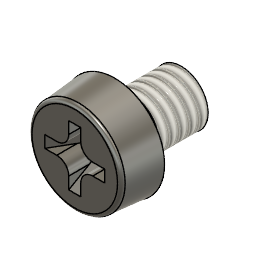
newest macropad desing (Autodesk Fusion 360 archive; units mm, degrees)
design "Cheese Head Screw BS EN ISO 7048 - M2.5 x 3 - H Steel 4.6 Plain"
description: Cheese Head Screw BS EN ISO 7048 - M2.5 x 3 - H
part number: BS EN ISO 7048 - H - M2.5 x 3 Steel 4.6 Plain
Autodesk Fusion 360 part; units mm, degrees
sketch "Sketch1" plane through (0, 0, 0) normal (0, 1, 0) x (1, 0, 0)
  line L0 (0, -1.8) -> (0, 3)
  line L1 (-2.25, 0) -> (-2.0925, -1.8)
  line L2 (-2.25, 0) -> (-1.0925, 0)
  line L3 (0, 3) -> (-1.25, 3)
  line L4 (-1.25, 3) -> (-1.25, 0.9)
  line L5 (-1.25, 0.9) -> (-1.0925, 0.3122)
  line L6 (-1.0925, 0.3122) -> (-1.0925, 0)
  line L7 (0, -1.8) -> (-2.0925, -1.8)
  dimension "d13" = 5
  dimension "d14" = 4.5
  dimension "d18" = 2.5
  dimension "d56" = 3
  dimension "d65" = 15
  dimension "d67" = 1.8
  dimension "d71" = 2.185
  dimension "d77" = 0.9
  constraint vertical L0
  constraint coincident origin L0
  constraint coincident origin L2
  constraint perpendicular L0 L3
  constraint coincident L2.end L6.end
  constraint perpendicular L0 L7
  measures "d13" angle of L0 L1
  measures "d56" distance of L2 L3
  measures "d65" angle of L5 L6
  measures "d67" distance of L1.start L7
  measures "d77" distance of L2 L4.end
revolve "Revolve1" add sketch "Sketch1" angle 360 about axis through (0, 0, 1.8) along (0, 0, -1) makes body 1
fillet "Fillet3" radius 0.18 1 edges at (-1.9509, 0.7567, 1.8) on bodies 1
fillet "Fillet2" radius 0.1 1 edges at (-1.0186, 0.3951, 0) on bodies 1
sketch "Sketch2" plane through (0, 0, 1.8) normal (0, 0, 1) x (1, 0, 0)
  line L0 (-0.27, 0.27) -> (-1.35, 0.27)
  line L1 (-1.35, 0.27) -> (-1.35, -0.27)
  line L2 (-1.35, -0.27) -> (-0.27, -0.27)
  line L3 (-0.27, -0.27) -> (-0.27, -1.35)
  line L4 (-0.27, -1.35) -> (0.27, -1.35)
  line L5 (0.27, -1.35) -> (0.27, -0.27)
  line L6 (0.27, -0.27) -> (1.35, -0.27)
  line L7 (1.35, -0.27) -> (1.35, 0.27)
  line L8 (1.35, 0.27) -> (0.27, 0.27)
  line L9 (0.27, 0.27) -> (0.27, 1.35)
  line L10 (0.27, 1.35) -> (-0.27, 1.35)
  line L11 (-0.27, 1.35) -> (-0.27, 0.27)
  dimension "d81" = 360
  dimension "d83" = 0.54
  dimension "d84" = 2.7
  constraint horizontal L0
  constraint perpendicular L0 L1
  constraint vertical L0.start L2.end
  constraint coincident L2.end L3.start
  measures "d83" distance of L0 L2
  measures "d84" distance of L1 L6.end
extrude "Extrude1" add sketch "Sketch2" against normal blind 1.2 separate body makes body 2
draft "Draft1" angle -30 neutral plane through (0, 0, 1.8) pull (0, 0, 1) 4 faces at (1.35, 0.09, 1) (0.09, 1.35, 1.4) (-1.35, 0.09, 1.4) (-0.09, -1.35, 1.4) on bodies 2
fillet "Fillet1" radius 0.54 4 edges at (-0.27, 0.27, 1.2) (-0.27, -0.27, 1.2) (0.27, -0.27, 1.2) (0.27, 0.27, 1.2) on bodies 2
combine "Combine1" operation cut target body 1 tool bodies 2
thread "Thread3" "ISO Metric profile 2.5 M2.5x0.45 M2.5x0.45 6g" major diameter 2.43 minor diameter 1.9165 pitch 0.45 angle 60 resizes the face on face at (-1.2484, -0.0623, -2.3) on bodies 1
equation "adsk_nomdia = 2.50 mm"
equation "adsk_nomlen = 3.00 mm"
equation "adsk_headdia = 4.50 mm"
equation "adsk_phildia = 2.70 mm"
equation "adsk_midfillet = 0.10 mm"
equation "adsk_phildepth = 1.20 mm"
equation "adsk_shnklen = 0.90 mm"
equation "adsk_thrang = 15 deg"
equation "adsk_headang = 5 deg"
equation "d13 = adsk_headang"
equation "d14 = adsk_headdia"
equation "d18 = adsk_nomdia"
equation "adsk_philwidth = 0.54 mm"
equation "d43 = -adsk_phildepth"
equation "d52 = adsk_midfillet"
equation "d56 = adsk_nomlen"
equation "d65 = adsk_thrang"
equation "d67 = adsk_headh"
equation "adsk_headh = 1.80 mm"
equation "adsk_pitch1 = 0.45 mm"
equation "adsk_shnkdia = adsk_nomdia - 0.7 * adsk_pitch1"
equation "d71 = adsk_shnkdia"
equation "adsk_headtoprad = adsk_headh * 0.1"
equation "d76 = adsk_headtoprad"
equation "d77 = adsk_shnklen"
equation "d83 = adsk_philwidth"
equation "d84 = adsk_phildia"
equation "d86 = adsk_philwidth"
